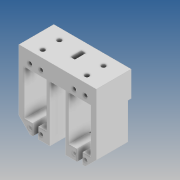
# Autodesk Inventor part: MotorBracket
Saved by Autodesk Inventor 2020 (Build 240168000, 168)
## iProperties
Created: 2019-08-15
Part Number: MotorBracket
Material: 일반
Document SubType Name: Modeling
Designer: Jeong Ji Hoon
Density: 1 g/cm^3
Appearance: 기본값
Author: Jeong Ji Hoon
## iProperties of the stored document _3D 인쇄.ipt
Created: 2019-08-15
Part Number: _3D 인쇄
Material: 일반
Document SubType Name: Modeling
Designer: Jeong Ji Hoon
Density: 1 g/cm^3
Appearance: 기본값
Author: Jeong Ji Hoon
Autodesk Inventor part; units mm, degrees
ref_plane "YZ Plane" through (0, 0, 0) normal (1, 0, 0) x (0, 1, 0)
ref_plane "XZ Plane" through (0, 0, 0) normal (0, 1, 0) x (-1, 0, 0)
ref_plane "XY Plane" through (0, 0, 0) normal (0, 0, 1) x (1, 0, 0)
sketch "스케치1" plane through (0, 0, 0) normal (0, 0, 1) x (1, 0, 0)
  line L0 (0, 0) -> (70, 0)
  line L1 (70, 0) -> (70, 65.5)
  line L2 (70, 65.5) -> (0, 65.5)
  line L3 (0, 65.5) -> (0, 0)
  line L4 (5, 50.5) -> (25, 50.5)
  line L5 (25, 50.5) -> (25, 10)
  line L6 (25, 10) -> (5, 10)
  line L7 (5, 10) -> (5, 50.5)
  line L8 (45, 50.5) -> (65, 50.5)
  line L9 (65, 50.5) -> (65, 10)
  line L10 (65, 10) -> (45, 10)
  line L11 (45, 10) -> (45, 50.5)
  line L12 (28, 50.5) -> (42, 50.5)
  line L13 (42, 50.5) -> (42, 0)
  line L14 (42, 0) -> (28, 0)
  line L15 (28, 0) -> (28, 50.5)
  line L16 (12.5, 10) -> (17.5, 10)
  line L17 (17.5, 10) -> (17.5, 0)
  line L18 (17.5, 0) -> (12.5, 0)
  line L19 (12.5, 0) -> (12.5, 10)
  line L20 (52.5, 10) -> (57.5, 10)
  line L21 (57.5, 10) -> (57.5, 0)
  line L22 (57.5, 0) -> (52.5, 0)
  line L23 (52.5, 0) -> (52.5, 10)
  point P0 (10, 5)
  point P1 (20, 5)
  point P2 (50, 5)
  point P3 (60, 5)
  point P4 (10, 55.5)
  point P5 (20, 55.5)
  point P6 (50, 55.5)
  point P7 (60, 55.5)
  dimension "d0" = 20
  dimension "d1" = 40.5
  dimension "d2" = 20
  dimension "d3" = 5
  dimension "d4" = 5
  dimension "d5" = 5
  dimension "d6" = 5
  dimension "d7" = 5
  dimension "d8" = 5
  dimension "d9" = 5
  dimension "d10" = 5
  dimension "d11" = 10
  dimension "d12" = 15
  dimension "d15" = 3
  dimension "d16" = 3
  dimension "d26" = 5
  dimension "d27" = 5
  dimension "d28" = 2.5
  dimension "d29" = 2.5
  constraints: 48 end point, 12 parallel, 6 horizontal, 6 horizontal alignment, 6 perpendicular, 5 point on line, 4 collinear, 4 vertical alignment
  measures "d0" distance of L5.end L6.end
  measures "d1" distance of L6.end L4.start
  measures "d2" distance between parallel lines of L11 L5
  measures "d3" distance between parallel lines of L3 L7
  measures "d4" distance between parallel lines of L1 L9
  measures "d5" distance from line of L7 point (10, 5)
  measures "d6" distance from line of point (20, 5) L5
  measures "d7" distance from line of L11 point (50, 5)
  measures "d8" distance from line of point (60, 5) L9
  measures "d9" distance from line of L6 point (10, 5)
  measures "d10" distance from line of point (10, 55.5) L4
  measures "d11" distance between parallel lines of L0 L6
  measures "d12" distance between parallel lines of L2 L4
  measures "d15" distance between parallel lines of L5 L15
  measures "d16" distance between parallel lines of L11 L13
  measures "d26" distance between parallel lines of L17 L19
  measures "d27" distance between parallel lines of L21 L23
  measures "d28" distance from line of point (10, 5) L19
  measures "d29" distance from line of point (50, 5) L23
extrude "돌출1" add sketch "스케치1" along normal blind 28.5 contours L3 L2 L1 L0 L21 L10 L9 L8 L11 L23 L13 L12 L15 L17 L6 L5 L4 L7 L19
hole "구멍1" at (10, 5, 0) at (20, 5, 0) at (50, 5, 0) at (60, 5, 0) at (10, 55.5, 0) at (20, 55.5, 0) at (50, 55.5, 0) at (60, 55.5, 0) direction (0, 0, 1) diameter 3.5 end through all
sketch "스케치3" plane through (17.5, 0, 0) normal (0, -1, 0) x (1, 0, 0)
  line L0 (0, 0) -> (10.5, 0) projected
  line L1 (10.5, 0) -> (10.5, 28.5) projected
  line L2 (0, 0) -> (0, 28.5) projected
  line L3 (24.5, 0) -> (35, 0) projected
  line L4 (35, 0) -> (35, 28.5) projected
  line L5 (24.5, 28.5) -> (35, 28.5) projected
  line L6 (24.5, 0) -> (24.5, 28.5) projected
  line L7 (0, 10) -> (35, 10)
  line L8 (35, 10) -> (35, 5)
  line L9 (35, 5) -> (0, 5)
  line L10 (0, 5) -> (0, 10)
  point P0 (-17.5, 0)
  point P1 (24.5, 5)
  point P2 (24.5, 10)
  point P3 (0, 5)
  point P4 (10.5, 5)
  point P5 (10.5, 10)
  dimension "d30" = 5
  dimension "d31" = 5
  constraints: 8 end point, 2 parallel, 2 point on line, 1 horizontal, 1 perpendicular
  measures "d30" distance between parallel lines of L9 L0
  measures "d31" distance between parallel lines of L7 L9
extrude "돌출2" cut sketch "스케치3" against normal blind 10 contours L2 L7 L1 L9 | L6 L7 L4 L9
sketch "스케치4" plane through (28, 50.5, 0) normal (0, -1, 0) x (1, 0, 0)
  line L0 (0, 0) -> (14, 0) projected
  line L1 (14, 0) -> (14, 28.5) projected
  line L2 (0, 0) -> (0, 28.5) projected
  line L3 (5, 15) -> (9, 15)
  line L4 (9, 15) -> (9, 5)
  line L5 (9, 5) -> (5, 5)
  line L6 (5, 5) -> (5, 15)
  point P0 (-28, 0)
  dimension "d34" = 5
  dimension "d35" = 5
  dimension "d36" = 10
  dimension "d37" = 5
  constraints: 8 end point, 2 parallel, 1 horizontal, 1 perpendicular
  measures "d34" distance between parallel lines of L2 L6
  measures "d35" distance between parallel lines of L1 L4
  measures "d36" distance between parallel lines of L3 L5
  measures "d37" distance between parallel lines of L0 L5
extrude "돌출3" cut sketch "스케치4" against normal through all
sketch "스케치6" plane through (0, 0, 0) normal (0, 0, -1) x (-1, 0, 0)
  circle A0 centre (-50, 55.5) radius 1.75 projected
  circle A1 centre (-10, 55.5) radius 1.75 projected
  circle A2 centre (-20, 55.5) radius 1.75 projected
  circle A3 centre (-60, 55.5) radius 1.75 projected
  line L0 (-28, 0) -> (-28, 50.5) projected
  line L1 (-25, 50.5) -> (-25, 10) projected
  line L2 (-5, 50.5) -> (-25, 50.5) projected
  line L3 (-5, 10) -> (-5, 50.5) projected
  line L4 (0, 65.5) -> (0, 0) projected
  line L5 (-70, 65.5) -> (0, 65.5) projected
  line L6 (-70, 0) -> (-70, 65.5) projected
  line L7 (-65, 50.5) -> (-65, 10) projected
  line L8 (-45, 50.5) -> (-65, 50.5) projected
  line L9 (-45, 10) -> (-45, 50.5) projected
  line L10 (-42, 50.5) -> (-42, 0) projected
  line L11 (-28, 50.5) -> (-42, 50.5) projected
  line L12 (0, 65.5) -> (-70, 65.5)
  line L13 (-70, 65.5) -> (-70, 42.5)
  line L14 (-70, 42.5) -> (0, 42.5)
  line L15 (0, 42.5) -> (0, 65.5)
  point P0 (-28, 42.5)
  point P1 (-25, 42.5)
  point P2 (-5, 42.5)
  point P3 (0, 42.5)
  point P4 (-65, 42.5)
  point P5 (-45, 42.5)
  point P6 (-42, 42.5)
  dimension "d40" = 23
  constraints: 8 end point, 2 parallel, 1 horizontal, 1 perpendicular, 1 point on line
  measures "d40" distance between parallel lines of L14 L12
extrude "돌출4" add sketch "스케치6" along normal blind 3
sketch "스케치7" plane through (0, 65.5, 28.5) normal (0, 1, 0) x (1, 0, 0)
  line L0 (0, 31.5) -> (0, 0) projected
  line L1 (70, 31.5) -> (70, 0) projected
  line L2 (0, 31.5) -> (70, 31.5) projected
  point P0 (0, 28.5)
  point P1 (55, 6.5)
  point P2 (55, 21.5)
  point P3 (15, 6.5)
  point P4 (15, 21.5)
  dimension "d43" = 15
  dimension "d44" = 15
  dimension "d45" = 10
  dimension "d46" = 15
  constraints: 2 horizontal alignment, 2 vertical alignment
  measures "d43" distance from line of L1 point (55, 6.5)
  measures "d44" distance from line of L0 point (15, 6.5)
  measures "d45" distance from line of L2 point (55, 21.5)
  measures "d46" distance of point (55, 6.5) point (55, 21.5)
hole "구멍2" at (55, 65.5, 22) at (55, 65.5, 7) at (15, 65.5, 22) at (15, 65.5, 7) direction (0, -1, 0) diameter 4 end through all
sketch "스케치8" plane through (0, 0, 0) normal (0, 0, -1) x (-1, 0, 0)
  circle A0 centre (-60, 5) radius 1.75 projected
  line L0 (-65, 42.5) -> (-70, 42.5) projected
  line L1 (-70, 0) -> (-70, 42.5) projected
  line L2 (-57.5, 0) -> (-70, 0) projected
  line L3 (-57.5, 10) -> (-57.5, 0) projected
  line L4 (-65, 10) -> (-57.5, 10) projected
  line L5 (-65, 42.5) -> (-65, 10) projected
  line L6 (0, 0) -> (-70, 0)
  line L7 (-70, 0) -> (-70, 10)
  line L8 (-70, 10) -> (0, 10)
  line L9 (0, 10) -> (0, 0)
  line L10 (-65, 10) -> (-57.5, 10) projected
  circle A1 centre (-20, 5) radius 1.75 projected
  line L11 (-25, 42.5) -> (-28, 42.5) projected
  line L12 (-28, 0) -> (-28, 42.5) projected
  line L13 (-17.5, 0) -> (-28, 0) projected
  line L14 (-17.5, 10) -> (-17.5, 0) projected
  line L15 (-25, 10) -> (-17.5, 10) projected
  line L16 (-25, 42.5) -> (-25, 10) projected
  circle A2 centre (-50, 5) radius 1.75 projected
  line L17 (-42, 42.5) -> (-45, 42.5) projected
  line L18 (-45, 10) -> (-45, 42.5) projected
  line L19 (-52.5, 10) -> (-45, 10) projected
  line L20 (-52.5, 0) -> (-52.5, 10) projected
  line L21 (-42, 0) -> (-52.5, 0) projected
  line L22 (-42, 42.5) -> (-42, 0) projected
  line L23 (-28, 0) -> (-42, 0)
  line L24 (-42, 0) -> (-42, 10)
  line L25 (-42, 10) -> (-28, 10)
  line L26 (-28, 10) -> (-28, 0)
  line L27 (-42, 42.5) -> (-42, 0) projected
  line L28 (-28, 0) -> (-42, 0)
  line L29 (-42, 0) -> (-42, 20)
  line L30 (-42, 20) -> (-28, 20)
  line L31 (-28, 20) -> (-28, 0)
  point P0 (-28, 10)
  dimension "d62" = 20
  constraints: 24 end point, 6 parallel, 4 point on line, 3 horizontal, 3 perpendicular, 1 collinear
  measures "d62" distance between parallel lines of L6 L30
extrude "돌출5" add sketch "스케치8" against normal blind 5 contours L22 L8 L12 L6 | L22 L30 L12 L8
sketch "스케치9" plane through (0, 0, 0) normal (0, 0, -1) x (-1, 0, 0)
  line L0 (-17.5, 0) -> (-52.5, 0) projected
  line L1 (-37.5, 0) -> (-32.5, 0)
  line L2 (-32.5, 0) -> (-32.5, 10)
  line L3 (-32.5, 10) -> (-37.5, 10)
  line L4 (-37.5, 10) -> (-37.5, 0)
  point P0 (0, 0)
  point P1 (-35, 0)
  dimension "d56" = 5
  dimension "d63" = 10
  constraints: 8 end point, 2 midpoint, 2 parallel, 1 horizontal, 1 perpendicular, 1 point on line
  measures "d56" distance between parallel lines of L2 L4
  measures "d63" distance of L3.end L1.start
extrude "돌출6" add sketch "스케치9" along normal blind 30
chamfer "모따기1" distance 10 angle 45 2 edges at (0, 0, 14.25) (70, 0, 14.25)
chamfer "모따기2" distance 5 angle 45 2 edges at (37.5, 5, 0) (32.5, 5, 0)
equation "\"d4\" = d3"
equation "\"d16\" = d15"
equation "\"d35\" = d34"
